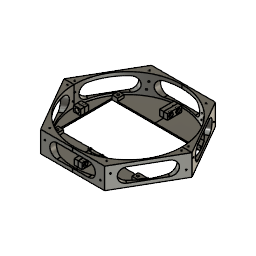
BoTech.StarClock.Top (Autodesk Fusion 360 design; units mm, degrees)
Autodesk Fusion 360 part; units mm, degrees
sketch "Skizze1" plane through (0, 0, 0) normal (0, 0, 1) x (1, 0, 0)
  line L0 (-60.5, 38) -> (60.5, 38)
  line L1 (60.5, 38) -> (60.5, -38)
  line L2 (60.5, -38) -> (-60.5, -38)
  line L3 (-60.5, -38) -> (-60.5, 38)
  line L4 (90, 0.0418) -> (44.9638, 77.9632)
  line L5 (44.9638, 77.9632) -> (-45.0362, 77.9214)
  line L6 (-45.0362, 77.9214) -> (-90, -0.0418)
  line L7 (-90, -0.0418) -> (-44.9638, -77.9632)
  line L8 (-44.9638, -77.9632) -> (45.0362, -77.9214)
  line L9 (45.0362, -77.9214) -> (90, 0.0418)
  line L10 (-0.0205, 160) -> (-138.5743, 79.9822)
  line L11 (-138.5743, 79.9822) -> (-138.5538, -80.0178)
  line L12 (-138.5538, -80.0178) -> (0.0205, -160)
  line L13 (0.0205, -160) -> (138.5743, -79.9822)
  line L14 (138.5743, -79.9822) -> (138.5538, 80.0178)
  line L15 (138.5538, 80.0178) -> (-0.0205, 160)
  line L16 (-45.0362, 77.9214) -> (-0.0205, 160)
  line L17 (-0.0205, 160) -> (44.9638, 77.9632)
  line L18 (44.9638, 77.9632) -> (138.5538, 80.0178)
  line L19 (138.5538, 80.0178) -> (90, 0.0418)
  line L20 (90, 0.0418) -> (138.5743, -79.9822)
  line L21 (138.5743, -79.9822) -> (45.0362, -77.9214)
  line L22 (-44.9638, -77.9632) -> (0.0205, -160)
  line L23 (0.0205, -160) -> (45.0362, -77.9214)
  line L24 (-90, -0.0418) -> (-138.5538, -80.0178)
  line L25 (-138.5538, -80.0178) -> (-44.9638, -77.9632)
  line L26 (-138.5743, 79.9822) -> (-90, -0.0418)
  line L27 (-45.0362, 77.9214) -> (-138.5743, 79.9822)
  circle A0 centre (0, 0) radius 75.8906
  circle A1 centre (-40, 70) radius 1
  circle A2 centre (-80, 5) radius 1
  circle A3 centre (-80, -5) radius 1
  circle A4 centre (40, 70) radius 1
  circle A5 centre (80, 5) radius 1
  circle A6 centre (80, -5) radius 1
  circle A7 centre (-40, -70) radius 1
  circle A8 centre (40, -70) radius 1
  circle A9 centre (0, -45) radius 4
  line L28 (4, -45) -> (6, -45)
  line L29 (-4, -45) -> (-6, -45)
  circle A10 centre (8.25, -45) radius 1
  circle A11 centre (8.25, -45) radius 2.25
  circle A12 centre (-8.2553, -45) radius 1
  circle A13 centre (-8.2553, -45) radius 2.25
  circle A14 centre (0, -45) radius 4
  line L30 (-4, -45) -> (-6, -45)
  line L31 (4, -45) -> (6, -45)
  line L32 (0, 0) -> (-60.5, 0)
  line L33 (-60.5, 0) -> (-60.5, 38)
  line L34 (60.5, -38) -> (52.5, -38)
  line L35 (52.5, -38) -> (52.5, -47)
  line L36 (52.5, -47) -> (60.5, -47)
  line L37 (60.5, -47) -> (60.5, -38)
  line L38 (-60.5, -38) -> (-52.5, -38)
  line L39 (-52.5, -38) -> (-52.5, -47)
  line L40 (-52.5, -47) -> (-60.5, -47)
  line L41 (-60.5, -47) -> (-60.5, -38)
  line L42 (60.5, 38) -> (52.5, 38)
  line L43 (52.5, 38) -> (52.5, 47)
  line L44 (52.5, 47) -> (60.5, 47)
  line L45 (60.5, 47) -> (60.5, 38)
  line L46 (-60.5, 38) -> (-52.5, 38)
  line L47 (-52.5, 38) -> (-52.5, 47)
  line L48 (-52.5, 47) -> (-60.5, 47)
  line L49 (-60.5, 47) -> (-60.5, 38)
  circle A15 centre (56.5, -42.5) radius 1.5
  line L50 (60.5, -38) -> (56.5, -38) construction
  line L51 (56.5, -38) -> (56.5, -42.5) construction
  line L52 (-52.5, -38) -> (-56.5, -38) construction
  line L53 (-56.5, -38) -> (-56.5, -42.5) construction
  circle A16 centre (-56.5, -42.5) radius 1.5
  line L54 (60.5, 47) -> (56.5, 47) construction
  line L55 (56.5, 47) -> (56.5, 42.5) construction
  line L56 (-52.5, 47) -> (-56.5, 47) construction
  line L57 (-56.5, 47) -> (-56.5, 42.5) construction
  circle A17 centre (56.5, 42.5) radius 1.5
  circle A18 centre (-56.5, 42.5) radius 1.5
  circle A19 centre (-56.5, -42.5) radius 2.75
  circle A20 centre (56.5, -42.5) radius 2.75
  circle A21 centre (56.5, 42.5) radius 2.75
  circle A22 centre (-56.5, 42.5) radius 2.75
  line L58 (60.5, -38) -> (65.6915, -38)
  line L59 (60.5, 38) -> (65.6915, 38)
  dimension "d1" = 121
  dimension "d2" = 76
  dimension "d26" = 90
  dimension "d43" = 160
  dimension "d258" = 2
  dimension "d259" = 2
  dimension "d260" = 2
  dimension "d261" = 2
  dimension "d262" = 2
  dimension "d263" = 2
  dimension "d264" = 2
  dimension "d265" = 2
  dimension "d322" = 8
  dimension "d323" = 2
  dimension "d324" = 2
  dimension "d325" = 2
  dimension "d326" = 4.5
  dimension "d327" = 2
  dimension "d328" = 4.5
  dimension "d331" = 8
  dimension "d332" = 2
  dimension "d333" = 2
  dimension "d350" = 60.5
  dimension "d351" = 38
  dimension "d352" = 8
  dimension "d353" = 9
  dimension "d354" = 8
  dimension "d355" = 9
  dimension "d356" = 8
  dimension "d357" = 9
  dimension "d358" = 8
  dimension "d359" = 9
  dimension "d362" = 3
  dimension "d363" = 4
  dimension "d364" = 4.5
  dimension "d365" = 4
  dimension "d366" = 4.5
  dimension "d367" = 3
  dimension "d368" = 4
  dimension "d369" = 4.5
  dimension "d370" = 4
  dimension "d371" = 4.5
  dimension "d372" = 3
  dimension "d373" = 3
  dimension "d376" = 5.5
  dimension "d377" = 5.5
  dimension "d378" = 5.5
  dimension "d379" = 5.5
  constraint horizontal L0
  constraint vertical L1
  constraint horizontal L2
  constraint vertical L3
  constraint coincident A0.centre L32.start
  constraint coincident A9 L28.start
  constraint parallel L2 L28
  constraint coincident A9 L29.start
  constraint parallel L2 L29
  constraint concentric A10 A11
  constraint coincident L28.end A11
  constraint concentric A12 A13
  constraint coincident L28.start A14
  constraint coincident L29.start A14
  constraint perpendicular L3 L32
  constraint perpendicular L32 L33
  constraint horizontal L34
  constraint vertical L35
  constraint horizontal L36
  constraint vertical L37
  constraint horizontal L38
  constraint vertical L39
  constraint horizontal L40
  constraint vertical L41
  constraint horizontal L42
  constraint vertical L43
  constraint horizontal L44
  constraint vertical L45
  constraint horizontal L46
  constraint vertical L47
  constraint horizontal L48
  constraint vertical L49
  constraint midpoint L34 L50.end
  constraint coincident A15.centre L51.end
  constraint coincident L53.end A16.centre
  constraint coincident L55.end A17.centre
  constraint coincident L57.end A18.centre
  constraint concentric A16 A19
  constraint concentric A15 A20
  constraint concentric A17 A21
  constraint concentric A18 A22
  constraint perpendicular L1 L58
  constraint coincident A0 L58.end
  constraint perpendicular L45 L59
  constraint coincident A0 L59.end
  measures "d1" distance of L0.end L0.start
  measures "d2" distance of L2.end L0.start
  measures "d26" distance of L4.start A0.centre
  measures "d43" distance of L10.start A0.centre
  measures "d258" diameter of A1
  measures "d259" diameter of A2
  measures "d260" diameter of A3
  measures "d261" diameter of A4
  measures "d262" diameter of A5
  measures "d263" diameter of A6
  measures "d264" diameter of A7
  measures "d265" diameter of A8
  measures "d322" diameter of A9
  measures "d323" distance of L28.start L28.end
  measures "d324" distance of L29.start L29.end
  measures "d325" diameter of A10
  measures "d326" diameter of A11
  measures "d327" diameter of A12
  measures "d328" diameter of A13
  measures "d331" diameter of A14
  measures "d332" distance of L28.start L28.end
  measures "d333" distance of L29.end L29.start
  measures "d350" distance of A0.centre L32.end
  measures "d351" distance of L32.end L0.start
  measures "d352" distance of L1.end L34.end
  measures "d353" distance of L1.end L36.end
  measures "d354" distance of L2.end L38.end
  measures "d355" distance of L2.end L40.end
  measures "d356" distance of L0.end L42.end
  measures "d357" distance of L0.end L44.end
  measures "d358" distance of L0.start L46.end
  measures "d359" distance of L0.start L48.end
  measures "d362" diameter of A15
  measures "d363" distance of L1.end L50.end
  measures "d364" distance of L50.end A15.centre
  measures "d365" distance of L38.end L52.end
  measures "d366" distance of L53.end L52.end
  measures "d367" diameter of A16
  measures "d368" distance of L44.end L54.end
  measures "d369" distance of L55.end L54.end
  measures "d370" distance of L47.end L56.end
  measures "d371" distance of L57.end L56.end
  measures "d372" diameter of A17
  measures "d373" diameter of A18
  measures "d376" diameter of A19
  measures "d377" diameter of A20
  measures "d378" diameter of A21
  measures "d379" diameter of A22
extrude "Extrusion1" add sketch "Skizze1" along normal blind 30 contours A0 L48 L49 | A0 L40 L41 | A0 L44 L45 | A0 L36 L37 | L4 L5 L6 L7 L8 L9 makes body 1
extrude "Extrusion2" add sketch "Skizze1" along normal blind 2 contours L0 A0 L46 L47 L48 L49 | L3 A0 L33 L41 L49 | L0 A0 L43 L44 L47 L48 | L0 A0 L42 L43 L44 L45 | L2 A0 L38 L39 L40 L41 | A0 L45 L59 | L2 A0 L35 L36 L39 L40 | L2 A0 L34 L35 L36 L37 | A0 L37 L58 | A1 | A2 | A3 | A4 | A5 | A6 | A7 | A8 | A10 | A11 | A12 | A13 | A19 | A20 | A21 | A22 bodies 1
extrude "Extrusion27" add sketch "Skizze1" along normal blind 8 contours A11 | A13 bodies 1
sketch "Skizze2" plane through (0.0362, -77.9423, 0) normal (0.000464, -1, 0) x (1, 0.000464, 0)
  line L0 (-45, 0) -> (45, 0)
  line L1 (45, 0) -> (45, 30)
  line L2 (-45, 30) -> (-45, 0)
  line L3 (-22, 25) -> (22, 25)
  line L4 (22, 25) -> (22, 5)
  line L5 (22, 5) -> (-22, 5)
  arc A0 (-22, 25) -> (-22, 5) centre (-22, 15) ccw
  arc A1 (22, 5) -> (22, 25) centre (22, 15) ccw
  circle A2 centre (39, 10) radius 3.5
  circle A3 centre (39, 10) radius 1
  circle A4 centre (39, 10) radius 2.5
  line L6 (-45, 30) -> (45, 30)
  line L7 (45, 30) -> (45, 0)
  line L8 (45, 0) -> (-45, 0)
  line L9 (-45, 0) -> (-45, 30)
  line L10 (45, 15) -> (39, 15)
  line L11 (39, 15) -> (22, 15)
  line L12 (22, 15) -> (-22, 15)
  line L13 (-22, 15) -> (-39, 15)
  line L14 (-39, 15) -> (-45, 15)
  circle A5 centre (-39, 20) radius 3.5
  circle A6 centre (-39, 20) radius 1
  circle A7 centre (-39, 20) radius 2.5
  line L15 (-39, 15) -> (-39, 20)
  line L16 (39, 15) -> (39, 10)
  point P0 (-57.5, 15)
  point P1 (-39, 20)
  dimension "d109" = 2
  dimension "d110" = 5
  dimension "d111" = 6
  dimension "d112" = 17
  dimension "d113" = 44
  dimension "d114" = 17
  dimension "d115" = 6
  dimension "d161" = 2
  dimension "d162" = 5
  dimension "d163" = 5
  dimension "d165" = 5
  constraint perpendicular L4 L5
  constraint tangent L3 A0
  constraint tangent L5 A1
  constraint concentric A3 A4
  constraint concentric A2 A4
  constraint horizontal L6
  constraint vertical L7
  constraint horizontal L8
  constraint vertical L9
  constraint coincident L0.end L1.start
  constraint coincident L2.start L6.start
  constraint midpoint L7 L10.start
  constraint perpendicular L7 L10
  constraint parallel L10 L11
  constraint perpendicular L4 L12
  constraint perpendicular L9 L14
  constraint concentric A6 A7
  constraint concentric A5 A7
  constraint coincident P1 A5.centre
  constraint perpendicular L13 L15
  constraint perpendicular L10 L16
  constraint coincident A2.centre A3.centre
  measures "d109" diameter of A3
  measures "d110" diameter of A4
  measures "d111" distance of L10.start L10.end
  measures "d112" distance of L10.end A1.centre
  measures "d113" distance of A1.centre A0.centre
  measures "d114" distance of A0.centre L13.end
  measures "d115" distance of L13.end L14.end
  measures "d161" diameter of A6
  measures "d162" diameter of A7
  measures "d163" distance of L13.end P1
  measures "d165" distance of L10.end A2.centre
sketch "Skizze3" plane through (67.5181, -38.9398, 0) normal (0.866257, -0.499598, 0) x (0.499598, 0.866257, 0)
  circle A0 centre (-39, 20) radius 3.5
  line L0 (22, 15) -> (-22, 15)
  circle A1 centre (-39, 20) radius 2.5
  line L1 (22, 5) -> (-22, 5)
  line L2 (-22, 25) -> (22, 25)
  line L3 (45, 0) -> (45, 30)
  line L4 (-39, 15) -> (-45, 15)
  line L5 (22, 25) -> (22, 5)
  line L6 (-45, 0) -> (-45, 30)
  line L7 (-45, 30) -> (-45, 0)
  line L8 (-45, 0) -> (45, 0)
  line L9 (-22, 15) -> (-39, 15)
  line L10 (-45, 30) -> (45, 30)
  line L11 (39, 15) -> (22, 15)
  line L12 (45, 30) -> (45, 0)
  line L13 (-39, 15) -> (-39, 20)
  arc A2 (22, 5) -> (22, 25) centre (22, 15) ccw
  circle A3 centre (-39, 20) radius 1
  circle A4 centre (39, 10) radius 3.5
  line L14 (45, 15) -> (39, 15)
  line L15 (39, 15) -> (39, 10)
  circle A5 centre (39, 10) radius 2.5
  line L16 (45, 0) -> (-45, 0)
  circle A6 centre (39, 10) radius 1
  arc A7 (-22, 25) -> (-22, 5) centre (-22, 15) ccw
  point P0 (-39, 20)
  dimension "d166" = 2
  dimension "d167" = 5
  dimension "d168" = 6
  dimension "d169" = 17
  dimension "d170" = 44
  dimension "d171" = 17
  dimension "d172" = 6
  dimension "d173" = 2
  dimension "d174" = 5
  dimension "d175" = 5
  dimension "d176" = 5
  constraint perpendicular L1 L5
  constraint tangent L2 A7
  constraint tangent L1 A2
  constraint concentric A5 A6
  constraint concentric A4 A5
  constraint horizontal L10
  constraint vertical L12
  constraint horizontal L16
  constraint vertical L6
  constraint coincident L3.start L8.end
  constraint coincident L6.end L7.start
  constraint midpoint L14.start L12
  constraint perpendicular L12 L14
  constraint parallel L11 L14
  constraint perpendicular L0 L5
  constraint perpendicular L4 L6
  constraint concentric A1 A3
  constraint concentric A0 A1
  constraint coincident P0 A0.centre
  constraint perpendicular L9 L13
  constraint perpendicular L14 L15
  constraint coincident A4.centre L15.end
  measures "d166" diameter of A6
  measures "d167" diameter of A5
  measures "d168" distance of L11.start L14.start
  measures "d169" distance of L0.start L11.start
  measures "d170" distance of L0.start L0.end
  measures "d171" distance of L0.end L4.start
  measures "d172" distance of L4.end L4.start
  measures "d173" diameter of A3
  measures "d174" diameter of A1
  measures "d175" distance of P0 L4.start
  measures "d176" distance of L11.start A4.centre
sketch "Skizze4" plane through (67.4819, 39.0025, 0) normal (0.865793, 0.500402, 0) x (-0.500402, 0.865793, 0)
  circle A0 centre (-39, 20) radius 3.5
  line L0 (22, 15) -> (-22, 15)
  circle A1 centre (-39, 20) radius 2.5
  line L1 (22, 5) -> (-22, 5)
  line L2 (-22, 25) -> (22, 25)
  line L3 (45, 0) -> (45, 30)
  line L4 (-39, 15) -> (-45, 15)
  line L5 (22, 25) -> (22, 5)
  line L6 (-45, 0) -> (-45, 30)
  line L7 (-45, 30) -> (-45, 0)
  line L8 (-45, 0) -> (45, 0)
  line L9 (-22, 15) -> (-39, 15)
  line L10 (-45, 30) -> (45, 30)
  line L11 (39, 15) -> (22, 15)
  line L12 (45, 30) -> (45, 0)
  line L13 (-39, 15) -> (-39, 20)
  arc A2 (22, 5) -> (22, 25) centre (22, 15) ccw
  circle A3 centre (-39, 20) radius 1
  circle A4 centre (39, 10) radius 3.5
  line L14 (45, 15) -> (39, 15)
  line L15 (39, 15) -> (39, 10)
  circle A5 centre (39, 10) radius 2.5
  line L16 (45, 0) -> (-45, 0)
  circle A6 centre (39, 10) radius 1
  arc A7 (-22, 25) -> (-22, 5) centre (-22, 15) ccw
  point P0 (-39, 20)
  dimension "d177" = 2
  dimension "d178" = 5
  dimension "d179" = 6
  dimension "d180" = 17
  dimension "d181" = 44
  dimension "d182" = 17
  dimension "d183" = 6
  dimension "d184" = 2
  dimension "d185" = 5
  dimension "d186" = 5
  dimension "d187" = 5
  constraint perpendicular L1 L5
  constraint tangent L2 A7
  constraint tangent L1 A2
  constraint concentric A5 A6
  constraint concentric A4 A5
  constraint horizontal L10
  constraint vertical L12
  constraint horizontal L16
  constraint vertical L6
  constraint coincident L3.start L8.end
  constraint coincident L6.end L7.start
  constraint midpoint L14.start L12
  constraint perpendicular L12 L14
  constraint parallel L11 L14
  constraint perpendicular L0 L5
  constraint perpendicular L4 L6
  constraint concentric A1 A3
  constraint concentric A0 A1
  constraint coincident P0 A0.centre
  constraint perpendicular L9 L13
  constraint perpendicular L14 L15
  constraint coincident A4.centre L15.end
  measures "d177" diameter of A6
  measures "d178" diameter of A5
  measures "d179" distance of L11.start L14.start
  measures "d180" distance of L0.start L11.start
  measures "d181" distance of L0.start L0.end
  measures "d182" distance of L0.end L4.start
  measures "d183" distance of L4.end L4.start
  measures "d184" diameter of A3
  measures "d185" diameter of A1
  measures "d186" distance of P0 L4.start
  measures "d187" distance of L11.start A4.centre
sketch "Skizze5" plane through (-0.0362, 77.9423, 0) normal (-0.000464, 1, 0) x (-1, -0.000464, 0)
  circle A0 centre (-39, 20) radius 3.5
  line L0 (22, 15) -> (-22, 15)
  circle A1 centre (-39, 20) radius 2.5
  line L1 (22, 5) -> (-22, 5)
  line L2 (-22, 25) -> (22, 25)
  line L3 (45, 0) -> (45, 30)
  line L4 (-39, 15) -> (-45, 15)
  line L5 (22, 25) -> (22, 5)
  line L6 (-45, 0) -> (-45, 30)
  line L7 (-45, 30) -> (-45, 0)
  line L8 (-45, 0) -> (45, 0)
  line L9 (-22, 15) -> (-39, 15)
  line L10 (-45, 30) -> (45, 30)
  line L11 (39, 15) -> (22, 15)
  line L12 (45, 30) -> (45, 0)
  line L13 (-39, 15) -> (-39, 20)
  arc A2 (22, 5) -> (22, 25) centre (22, 15) ccw
  circle A3 centre (-39, 20) radius 1
  circle A4 centre (39, 10) radius 3.5
  line L14 (45, 15) -> (39, 15)
  line L15 (39, 15) -> (39, 10)
  circle A5 centre (39, 10) radius 2.5
  line L16 (45, 0) -> (-45, 0)
  circle A6 centre (39, 10) radius 1
  arc A7 (-22, 25) -> (-22, 5) centre (-22, 15) ccw
  point P0 (-39, 20)
  dimension "d188" = 2
  dimension "d189" = 5
  dimension "d190" = 6
  dimension "d191" = 17
  dimension "d192" = 44
  dimension "d193" = 17
  dimension "d194" = 6
  dimension "d195" = 2
  dimension "d196" = 5
  dimension "d197" = 5
  dimension "d198" = 5
  constraint perpendicular L1 L5
  constraint tangent L2 A7
  constraint tangent L1 A2
  constraint concentric A5 A6
  constraint concentric A4 A5
  constraint horizontal L10
  constraint vertical L12
  constraint horizontal L16
  constraint vertical L6
  constraint coincident L3.start L8.end
  constraint coincident L6.end L7.start
  constraint midpoint L14.start L12
  constraint perpendicular L12 L14
  constraint parallel L11 L14
  constraint perpendicular L0 L5
  constraint perpendicular L4 L6
  constraint concentric A1 A3
  constraint concentric A0 A1
  constraint coincident P0 A0.centre
  constraint perpendicular L9 L13
  constraint perpendicular L14 L15
  constraint coincident A4.centre L15.end
  measures "d188" diameter of A6
  measures "d189" diameter of A5
  measures "d190" distance of L11.start L14.start
  measures "d191" distance of L0.start L11.start
  measures "d192" distance of L0.start L0.end
  measures "d193" distance of L0.end L4.start
  measures "d194" distance of L4.end L4.start
  measures "d195" diameter of A3
  measures "d196" diameter of A1
  measures "d197" distance of P0 L4.start
  measures "d198" distance of L11.start A4.centre
sketch "Skizze6" plane through (-67.5181, 38.9398, 0) normal (-0.866257, 0.499598, 0) x (-0.499598, -0.866257, 0)
  circle A0 centre (-39, 20) radius 3.5
  line L0 (22, 15) -> (-22, 15)
  circle A1 centre (-39, 20) radius 2.5
  line L1 (22, 5) -> (-22, 5)
  line L2 (-22, 25) -> (22, 25)
  line L3 (45, 0) -> (45, 30)
  line L4 (-39, 15) -> (-45, 15)
  line L5 (22, 25) -> (22, 5)
  line L6 (-45, 0) -> (-45, 30)
  line L7 (-45, 30) -> (-45, 0)
  line L8 (-45, 0) -> (45, 0)
  line L9 (-22, 15) -> (-39, 15)
  line L10 (-45, 30) -> (45, 30)
  line L11 (39, 15) -> (22, 15)
  line L12 (45, 30) -> (45, 0)
  line L13 (-39, 15) -> (-39, 20)
  arc A2 (22, 5) -> (22, 25) centre (22, 15) ccw
  circle A3 centre (-39, 20) radius 1
  circle A4 centre (39, 10) radius 3.5
  line L14 (45, 15) -> (39, 15)
  line L15 (39, 15) -> (39, 10)
  circle A5 centre (39, 10) radius 2.5
  line L16 (45, 0) -> (-45, 0)
  circle A6 centre (39, 10) radius 1
  arc A7 (-22, 25) -> (-22, 5) centre (-22, 15) ccw
  point P0 (-39, 20)
  dimension "d199" = 2
  dimension "d200" = 5
  dimension "d201" = 6
  dimension "d202" = 17
  dimension "d203" = 44
  dimension "d204" = 17
  dimension "d205" = 6
  dimension "d206" = 2
  dimension "d207" = 5
  dimension "d208" = 5
  dimension "d209" = 5
  constraint perpendicular L1 L5
  constraint tangent L2 A7
  constraint tangent L1 A2
  constraint concentric A5 A6
  constraint concentric A4 A5
  constraint horizontal L10
  constraint vertical L12
  constraint horizontal L16
  constraint vertical L6
  constraint coincident L3.start L8.end
  constraint coincident L6.end L7.start
  constraint midpoint L14.start L12
  constraint perpendicular L12 L14
  constraint parallel L11 L14
  constraint perpendicular L0 L5
  constraint perpendicular L4 L6
  constraint concentric A1 A3
  constraint concentric A0 A1
  constraint coincident P0 A0.centre
  constraint perpendicular L9 L13
  constraint perpendicular L14 L15
  constraint coincident A4.centre L15.end
  measures "d199" diameter of A6
  measures "d200" diameter of A5
  measures "d201" distance of L11.start L14.start
  measures "d202" distance of L0.start L11.start
  measures "d203" distance of L0.start L0.end
  measures "d204" distance of L0.end L4.start
  measures "d205" distance of L4.end L4.start
  measures "d206" diameter of A3
  measures "d207" diameter of A1
  measures "d208" distance of P0 L4.start
  measures "d209" distance of L11.start A4.centre
sketch "Skizze7" plane through (-67.4819, -39.0025, 0) normal (-0.865793, -0.500402, 0) x (0.500402, -0.865793, 0)
  circle A0 centre (-39, 20) radius 3.5
  line L0 (22, 15) -> (-22, 15)
  circle A1 centre (-39, 20) radius 2.5
  line L1 (22, 5) -> (-22, 5)
  line L2 (-22, 25) -> (22, 25)
  line L3 (45, 0) -> (45, 30)
  line L4 (-39, 15) -> (-45, 15)
  line L5 (22, 25) -> (22, 5)
  line L6 (-45, 0) -> (-45, 30)
  line L7 (-45, 30) -> (-45, 0)
  line L8 (-45, 0) -> (45, 0)
  line L9 (-22, 15) -> (-39, 15)
  line L10 (-45, 30) -> (45, 30)
  line L11 (39, 15) -> (22, 15)
  line L12 (45, 30) -> (45, 0)
  line L13 (-39, 15) -> (-39, 20)
  arc A2 (22, 5) -> (22, 25) centre (22, 15) ccw
  circle A3 centre (-39, 20) radius 1
  circle A4 centre (39, 10) radius 3.5
  line L14 (45, 15) -> (39, 15)
  line L15 (39, 15) -> (39, 10)
  circle A5 centre (39, 10) radius 2.5
  line L16 (45, 0) -> (-45, 0)
  circle A6 centre (39, 10) radius 1
  arc A7 (-22, 25) -> (-22, 5) centre (-22, 15) ccw
  point P0 (-39, 20)
  dimension "d210" = 2
  dimension "d211" = 5
  dimension "d212" = 6
  dimension "d213" = 17
  dimension "d214" = 44
  dimension "d215" = 17
  dimension "d216" = 6
  dimension "d217" = 2
  dimension "d218" = 5
  dimension "d219" = 5
  dimension "d220" = 5
  constraint perpendicular L1 L5
  constraint tangent L2 A7
  constraint tangent L1 A2
  constraint concentric A5 A6
  constraint concentric A4 A5
  constraint horizontal L10
  constraint vertical L12
  constraint horizontal L16
  constraint vertical L6
  constraint coincident L3.start L8.end
  constraint coincident L6.end L7.start
  constraint midpoint L14.start L12
  constraint perpendicular L12 L14
  constraint parallel L11 L14
  constraint perpendicular L0 L5
  constraint perpendicular L4 L6
  constraint concentric A1 A3
  constraint concentric A0 A1
  constraint coincident P0 A0.centre
  constraint perpendicular L9 L13
  constraint perpendicular L14 L15
  constraint coincident A4.centre L15.end
  measures "d210" diameter of A6
  measures "d211" diameter of A5
  measures "d212" distance of L11.start L14.start
  measures "d213" distance of L0.start L11.start
  measures "d214" distance of L0.start L0.end
  measures "d215" distance of L0.end L4.start
  measures "d216" distance of L4.end L4.start
  measures "d217" diameter of A3
  measures "d218" diameter of A1
  measures "d219" distance of P0 L4.start
  measures "d220" distance of L11.start A4.centre
extrude "Extrusion3" cut sketch "Skizze2" against normal blind 28 contours L4 L5 A0 L12 L13 | L3 L4 A0 L12 L13 | L4 A1 L11 | L4 A1 L11 | A3 | A6 bodies 1
extrude "Extrusion4" cut sketch "Skizze7" against normal blind 28 contours L0 L1 L5 L9 A7 | L0 L2 L5 L9 A7 | L5 L11 A2 | L5 L11 A2 | A3 | A6 bodies 1
extrude "Extrusion5" cut sketch "Skizze6" against normal blind 28 contours L0 L1 L5 L9 A7 | L0 L2 L5 L9 A7 | L5 L11 A2 | L5 L11 A2 | A3 | A6 bodies 1
extrude "Extrusion6" cut sketch "Skizze5" against normal blind 28 contours L0 L1 L5 L9 A7 | L0 L2 L5 L9 A7 | L5 L11 A2 | L5 L11 A2 | A3 | A6 bodies 1
extrude "Extrusion7" cut sketch "Skizze4" against normal blind 28 contours L0 L1 L5 L9 A7 | L0 L2 L5 L9 A7 | L5 L11 A2 | L5 L11 A2 | A3 | A6 bodies 1
extrude "Extrusion8" cut sketch "Skizze3" against normal blind 28 contours L0 L1 L5 L9 A7 | L0 L2 L5 L9 A7 | L5 L11 A2 | L5 L11 A2 | A3 | A6 bodies 1
extrude "Extrusion28" cut sketch "Skizze1" along normal blind 3 from surface at 2 contours A0 L48 L49 | A0 L40 L41 | A0 L44 L45 | A0 L36 L37 bodies 1
extrude "Extrusion29" add sketch "Skizze1" along normal blind 6 contours L0 A0 L46 L47 L48 L49 | A0 L48 L49 | L0 A0 L42 L43 L44 L45 | L2 A0 L38 L39 L40 L41 | A0 L40 L41 | A0 L45 L59 | A0 L44 L45 | L2 A0 L34 L35 L36 L37 | A0 L37 L58 | A0 L36 L37 | A19 | A20 | A21 | A22 bodies 1
extrude "Extrusion30" cut sketch "Skizze1" along normal blind 4 contours A19 | A20 | A21 | A22 bodies 1
sketch "Skizze19" plane through (0, -38, 0) normal (0, 1, 0) x (-1, 0, 0)
  line L0 (-65.6915, 0) -> (60.5, 0)
  line L1 (60.5, 0) -> (60.5, 2)
  line L2 (60.5, 2) -> (60.5, 6)
  line L3 (60.5, 6) -> (52.5, 6)
  line L4 (52.5, 6) -> (52.5, 2)
  line L5 (52.5, 2) -> (-52.5, 2)
  line L6 (-52.5, 2) -> (-52.5, 6)
  line L7 (-52.5, 6) -> (-65.6915, 6)
  line L8 (-65.6915, 6) -> (-65.6915, 5)
  line L9 (-65.6915, 5) -> (-65.6915, 0)
  line L10 (-60.5, 0) -> (-60.5, 6)
  line L11 (-65.6915, 6) -> (-52.5, 6)
  line L12 (-52.5, 6) -> (-52.5, 0)
  line L13 (-52.5, 0) -> (-65.6915, 0)
  line L14 (-65.6915, 0) -> (-65.6915, 6)
  circle A0 centre (-63.0958, 3) radius 1
  line L15 (-60.5, 3) -> (-65.6915, 3)
  circle A1 centre (-63.0958, 3) radius 1.5
  line L16 (-61.5958, 3) -> (-61.0958, 3)
  line L17 (-63.0958, 4.5) -> (-63.0958, 5)
  line L18 (-61.1, 5) -> (-65.1, 5)
  line L19 (-65.1, 5) -> (-65.1, 1)
  line L20 (-65.1, 1) -> (-63, 1)
  line L21 (-61.1, 2.9) -> (-61.1, 5)
  arc A2 (-63, 1) -> (-61.1, 2.9) centre (-63, 2.9) ccw
  point P0 (-61.1, 1)
  dimension "d382" = 2
  dimension "d383" = 5.1915
  dimension "d386" = 3
  dimension "d387" = 0.5
  dimension "d388" = 0.5
  dimension "d389" = 4
  dimension "d390" = 4
  dimension "d391" = 1.9
  constraint coincident L0 L10.start
  constraint coincident L7 L10.end
  constraint perpendicular L7 L10
  constraint horizontal L11
  constraint vertical L12
  constraint horizontal L13
  constraint vertical L14
  constraint coincident L0 L12.end
  constraint coincident L7.end L8.start
  constraint midpoint L10 L15.start
  constraint midpoint L14 L15.end
  constraint midpoint A0.centre L15
  constraint concentric A0 A1
  constraint coincident L15 L16.start
  constraint coincident A1 L16.start
  constraint coincident L15 L16.end
  constraint coincident A1 L17.start
  constraint perpendicular L15 L17
  constraint horizontal L18
  constraint vertical L19
  constraint horizontal L20
  constraint vertical L21
  constraint coincident P0 L21
  constraint coincident P0 L20
  constraint tangent L21 A2
  constraint tangent L20 A2
  measures "d382" diameter of A0
  measures "d383" distance of L15.start L15.end
  measures "d386" diameter of A1
  measures "d387" distance of L16.start L16.end
  measures "d388" distance of L17.start L17.end
  measures "d389" distance of L18.start L18.end
  measures "d390" distance of L18.start P0
  measures "d391" radius of A2
extrude "Extrusion31" add sketch "Skizze19" along normal blind 3 contours A0 L15 | A0 L15 bodies 1
extrude "Extrusion32" add sketch "Skizze19" along normal blind 3 from surface at 73 contours A0 L15 | A0 L15 bodies 1
sketch "Skizze8" plane through (0, 0, 2) normal (0, 0, 1) x (-1, 0, 0)
  line L0 (0, -20) -> (0, 10)
  line L1 (5.5, 70) -> (-5.5, 70)
  line L2 (-5.5, 70) -> (-5.5, 50)
  line L3 (-5.5, 50) -> (5.5, 50)
  line L4 (5.5, 50) -> (5.5, 70)
  line L5 (15, -0.0337) -> (-20, -0.0337)
  line L6 (61, 5.5) -> (71, 5.5)
  line L7 (71, 5.5) -> (71, -5.5)
  line L8 (61, -5.5) -> (61, 5.5)
  line L9 (71, -5.5) -> (61, -5.5)
  line L10 (-45.0362, 77.9214) -> (-90, -0.0418)
  line L11 (-90, -0.0418) -> (-44.9638, -77.9632)
  line L12 (5.5, -70.0674) -> (-5.5, -70.0674)
  line L13 (-5.5, -70.0674) -> (-5.5, -50.0674)
  line L14 (5.5, -50.0674) -> (5.5, -70.0674)
  line L15 (-5.5, -50.0674) -> (5.5, -50.0674)
  circle A0 centre (-40, 70) radius 1
  circle A1 centre (40, -70) radius 1
  circle A2 centre (80, -5) radius 1
  circle A3 centre (-40, -70) radius 1
  circle A4 centre (40, 70) radius 1
  circle A5 centre (-80, 5) radius 1
  circle A6 centre (-8.25, 45) radius 1
  circle A7 centre (80, 5) radius 1
  circle A8 centre (-80, -5) radius 1
  circle A9 centre (8.2553, 45) radius 1
  dimension "d101" = 11
  dimension "d102" = 20
  constraint vertical L0
  constraint horizontal L1
  constraint vertical L2
  constraint horizontal L3
  constraint vertical L4
  constraint perpendicular L0 L5
  constraint symmetric L1.start L5 L12.start
  constraint symmetric L1.end L5 L12.end
  constraint symmetric L2.end L5 L13.end
  constraint symmetric L3.end L5 L14.start
  measures "d101" distance of L1.start L1.end
  measures "d102" distance of L1.start L3.end
extrude "Extrusion9" add sketch "Skizze8" along normal blind 8 contours L1 L2 L3 L4 | L6 L7 L8 L9 | L12 L13 L14 L15 bodies 1
sketch "Skizze11" plane through (0, -5.5, 0) normal (0, -1, 0) x (1, 0, 0)
  line L0 (-71, 2) -> (-61, 2)
  line L1 (-61, 2) -> (-61, 10)
  line L2 (-71, 10) -> (-71, 2)
  line L3 (0, 0) -> (0, 20)
  line L4 (71, 12) -> (71, 2)
  line L5 (71, 2) -> (61, 2)
  line L6 (61, 2) -> (61, 12)
  circle A0 centre (-66, 6) radius 3
  circle A1 centre (-66, 6) radius 1.75
  circle A2 centre (66, 6) radius 1.75
  circle A3 centre (66, 6) radius 3
  constraint coincident L3.start origin
  constraint vertical L3
  constraint symmetric L0.start L3 L4.end
  constraint symmetric L0.end L3 L5.end
  constraint coincident A0.centre A1.centre
  constraint symmetric L3 A0 A3
  constraint symmetric L3 A1 A2
sketch "Skizze12" plane through (-5.5, 0, 0) normal (-1, 0, 0) x (0, -1, 0)
  line L0 (-70.0674, 2) -> (-60.0674, 2)
  line L1 (-60.0674, 2) -> (-60.0674, 10)
  line L2 (-70.0674, 10) -> (-70.0674, 2)
  line L3 (0, 0) -> (0, 20)
  circle A0 centre (-65, 6) radius 3
  circle A1 centre (-65, 6) radius 1.75
  line L4 (-70.0674, 2) -> (-50.0674, 2)
  line L5 (-50.0674, 2) -> (-50.0674, 10)
  line L6 (-50.0674, 10) -> (-70.0674, 10)
  line L7 (-70.0674, 10) -> (-70.0674, 2)
  circle A2 centre (-55, 6) radius 3
  circle A3 centre (-55, 6) radius 1.75
  line L8 (70.0674, 2) -> (50.0674, 2)
  line L9 (50.0674, 2) -> (50.0674, 10)
  line L10 (70.0674, 10) -> (70.0674, 2)
  line L11 (70.0674, 2) -> (60.0674, 2)
  circle A4 centre (65, 6) radius 3
  line L12 (70.0674, 10) -> (70.0674, 2)
  circle A5 centre (55, 6) radius 3
  line L13 (50.0674, 10) -> (70.0674, 10)
  circle A6 centre (65, 6) radius 1.75
  line L14 (60.0674, 2) -> (60.0674, 10)
  circle A7 centre (55, 6) radius 1.75
  constraint coincident L3.start origin
  constraint vertical L3
  constraint symmetric L0.start L3 L8.start
  constraint symmetric L0.end L3 L11.end
  constraint symmetric L1.end L3 L14.end
  constraint symmetric L2.start L3 L10.start
  constraint symmetric L3 A0 A4
  constraint symmetric L3 A1 A6
  constraint symmetric L3 L0.start L8.start
  constraint symmetric L3 L4.end L8.end
  constraint symmetric L3 L5.end L9.end
  constraint symmetric L3 L2.start L10.start
  constraint symmetric L3 A2 A5
  constraint symmetric L3 A3 A7
sketch "Skizze13" plane through (5.5, 0, 0) normal (1, 0, 0) x (0, 1, 0)
  line L0 (60.0674, 2) -> (70.0674, 2)
  line L1 (70.0674, 2) -> (70.0674, 10)
  line L2 (70.0674, 10) -> (60.0674, 10)
  line L3 (60.0674, 10) -> (60.0674, 2)
  line L4 (66.7321, 3) -> (63.2679, 3)
  line L5 (68.4641, 6) -> (66.7321, 3)
  line L6 (66.7321, 9) -> (68.4641, 6)
  line L7 (63.2679, 3) -> (61.5359, 6)
  line L8 (61.5359, 6) -> (63.2679, 9)
  circle A0 centre (65, 6) radius 1.75
  line L9 (63.2679, 9) -> (66.7321, 9)
  line L10 (66.7321, 3) -> (63.2679, 3)
  line L11 (68.4641, 6) -> (66.7321, 3)
  line L12 (66.7321, 9) -> (68.4641, 6)
  line L13 (63.2679, 3) -> (61.5359, 6)
  line L14 (61.5359, 6) -> (63.2679, 9)
  circle A1 centre (65, 6) radius 1.75
  line L15 (63.2679, 9) -> (66.7321, 9)
  line L16 (0, 0) -> (0, 15.511)
  line L17 (50.0674, 2) -> (70.0674, 2)
  line L18 (70.0674, 2) -> (70.0674, 10)
  line L19 (70.0674, 10) -> (50.0674, 10)
  line L20 (50.0674, 10) -> (50.0674, 2)
  line L21 (58.4641, 6) -> (56.7321, 3)
  line L22 (53.2679, 9) -> (56.7321, 9)
  line L23 (56.7321, 3) -> (53.2679, 3)
  line L24 (53.2679, 3) -> (51.5359, 6)
  line L25 (53.2679, 9) -> (56.7321, 9)
  circle A2 centre (55, 6) radius 1.75
  line L26 (56.7321, 9) -> (58.4641, 6)
  line L27 (56.7321, 9) -> (58.4641, 6)
  circle A3 centre (55, 6) radius 1.75
  line L28 (56.7321, 3) -> (53.2679, 3)
  line L29 (58.4641, 6) -> (56.7321, 3)
  line L30 (53.2679, 3) -> (51.5359, 6)
  line L31 (51.5359, 6) -> (53.2679, 9)
  line L32 (51.5359, 6) -> (53.2679, 9)
  line L33 (-53.2679, 3) -> (-51.5359, 6)
  line L34 (-70.0674, 2) -> (-70.0674, 10)
  line L35 (-60.0674, 2) -> (-70.0674, 2)
  line L36 (-63.2679, 3) -> (-61.5359, 6)
  line L37 (-66.7321, 3) -> (-63.2679, 3)
  line L38 (-63.2679, 9) -> (-66.7321, 9)
  line L39 (-50.0674, 2) -> (-70.0674, 2)
  line L40 (-63.2679, 9) -> (-66.7321, 9)
  line L41 (-68.4641, 6) -> (-66.7321, 3)
  circle A4 centre (-55, 6) radius 1.75
  circle A5 centre (-55, 6) radius 1.75
  line L42 (-56.7321, 9) -> (-58.4641, 6)
  line L43 (-51.5359, 6) -> (-53.2679, 9)
  line L44 (-56.7321, 3) -> (-53.2679, 3)
  line L45 (-58.4641, 6) -> (-56.7321, 3)
  line L46 (-53.2679, 9) -> (-56.7321, 9)
  line L47 (-51.5359, 6) -> (-53.2679, 9)
  line L48 (-56.7321, 3) -> (-53.2679, 3)
  line L49 (-61.5359, 6) -> (-63.2679, 9)
  line L50 (-60.0674, 10) -> (-60.0674, 2)
  line L51 (-70.0674, 2) -> (-70.0674, 10)
  line L52 (-63.2679, 3) -> (-61.5359, 6)
  line L53 (-58.4641, 6) -> (-56.7321, 3)
  line L54 (-70.0674, 10) -> (-60.0674, 10)
  line L55 (-66.7321, 3) -> (-63.2679, 3)
  line L56 (-66.7321, 9) -> (-68.4641, 6)
  line L57 (-53.2679, 9) -> (-56.7321, 9)
  circle A6 centre (-65, 6) radius 1.75
  line L58 (-53.2679, 3) -> (-51.5359, 6)
  line L59 (-56.7321, 9) -> (-58.4641, 6)
  line L60 (-50.0674, 10) -> (-50.0674, 2)
  line L61 (-68.4641, 6) -> (-66.7321, 3)
  line L62 (-61.5359, 6) -> (-63.2679, 9)
  circle A7 centre (-65, 6) radius 1.75
  line L63 (-70.0674, 10) -> (-50.0674, 10)
  line L64 (-66.7321, 9) -> (-68.4641, 6)
  point P0 (65, 6)
  point P1 (65, 6)
  point P2 (55, 6)
  point P3 (55, 6)
  point P4 (-55, 6)
  point P5 (-55, 6)
  point P6 (-65, 6)
  point P7 (-65, 6)
  constraint coincident L16.start origin
  constraint vertical L16
  constraint symmetric L0.start L16 L35.start
  constraint symmetric L0.end L16 L34.start
  constraint symmetric L1.end L16 L34.end
  constraint symmetric L2.end L16 L50.start
  constraint symmetric L5.start L16 L41.start
  constraint symmetric L8.end L16 L38.start
  constraint symmetric P1 L16 P6
  constraint symmetric L6.start L16 L38.end
  constraint symmetric L4.end L16 L36.start
  constraint symmetric L4.start L16 L37.start
  constraint symmetric L7.end L16 L36.end
  constraint symmetric A0 L16 A7
  constraint symmetric P1 L16 P7
  constraint symmetric A1 L16 A6
  constraint symmetric L16 L17.start L39.start
  constraint symmetric L16 L0.end L34.start
  constraint symmetric L16 L1.end L34.end
  constraint symmetric L16 L19.end L60.start
  constraint symmetric L16 L21.end L44.start
  constraint symmetric L16 P3 P5
  constraint symmetric L16 L21.start L42.end
  constraint symmetric L16 L23.end L33.start
  constraint symmetric L16 L22.start L43.end
  constraint symmetric L16 L24.end L33.end
  constraint symmetric L16 L22.end L42.start
  constraint symmetric L16 A2 A5
  constraint symmetric L16 A3 A4
sketch "Skizze14" plane through (0, 5.5, 0) normal (0, 1, 0) x (-1, 0, 0)
  line L0 (61, 2) -> (71, 2)
  line L1 (71, 2) -> (71, 10)
  line L2 (71, 10) -> (61, 10)
  line L3 (61, 10) -> (61, 2)
  line L4 (67.7321, 3) -> (64.2679, 3)
  line L5 (69.4641, 6) -> (67.7321, 3)
  line L6 (67.7321, 9) -> (69.4641, 6)
  line L7 (64.2679, 3) -> (62.5359, 6)
  line L8 (62.5359, 6) -> (64.2679, 9)
  circle A0 centre (66, 6) radius 1.75
  line L9 (64.2679, 9) -> (67.7321, 9)
  line L10 (0, 0) -> (0, 20)
  line L11 (-64.2679, 9) -> (-67.7321, 9)
  line L12 (-67.7321, 3) -> (-64.2679, 3)
  line L13 (-62.5359, 6) -> (-64.2679, 9)
  line L14 (-67.7321, 9) -> (-69.4641, 6)
  line L15 (-64.2679, 3) -> (-62.5359, 6)
  circle A1 centre (-66, 6) radius 1.75
  line L16 (-69.4641, 6) -> (-67.7321, 3)
  point P0 (66, 6)
  point P1 (-66, 6)
  constraint symmetric L5.start L10 L14.end
  constraint symmetric L8.end L10 L11.start
  constraint symmetric P0 L10 P1
  constraint symmetric L6.start L10 L11.end
  constraint symmetric L4.end L10 L12.end
  constraint symmetric L4.start L10 L12.start
  constraint symmetric L7.end L10 L13.start
  constraint symmetric A0 L10 A1
extrude "Extrusion14" cut sketch "Skizze12" against normal blind 3.75 contours A0 | A1 | A2 | A3 | A4 | A5 | A6 | A7 bodies 1
extrude "Extrusion15" cut sketch "Skizze11" against normal blind 3.75 contours A0 | A1 bodies 1
extrude "Extrusion16" cut sketch "Skizze13" against normal blind 2.75 contours L4 L5 L6 L7 L8 L9 L10 L11 L12 L13 L14 L15 | A0 A1 | L21 L22 L23 L24 L25 L26 L27 L28 L29 L30 L31 L32 | A2 A3 | L33 L42 L43 L44 L45 L46 L47 L48 L53 L57 L58 L59 | L36 L37 L38 L40 L41 L49 L52 L55 L56 L61 L62 L64 | A4 A5 | A6 A7 bodies 1
extrude "Extrusion17" cut sketch "Skizze14" against normal blind 2.75 contours L4 L5 L6 L7 L8 L9 | A0 bodies 1
extrude "Extrusion18" cut sketch "Skizze14" against normal blind 11 contours A0 | A1 bodies 1
extrude "Extrusion19" cut sketch "Skizze13" against normal blind 11 contours A0 A1 | A2 A3 | A4 A5 | A6 A7 bodies 1
split "Teilen1" by plane through (0, 0, 0) normal (0, 1, 0) bodies 1 makes body 2 at (14.9879, 54.5943, 0)
split "Teilen2" by plane through (0, 0, 0) normal (1, 0, 0) bodies 1 2 makes body 4 at (32.9453, 53.0912, 0) makes body 3 at (34.2988, -55.9138, 0)
copy_body "Körper->Berechn3" bodies 2 removing the originals makes body 5 in component "BoTech.StarClock.Top.A"
copy_body "Körper->Berechn4" bodies 1 removing the originals makes body 6 in component "BoTech.StarClock.Top.B"
copy_body "Körper->Berechn5" bodies 3 removing the originals makes body 7 in component "BoTech.StarClock.Top.C"
copy_body "Körper->Berechn6" bodies 4 removing the originals makes body 8 in component "BoTech.StarClock.Top.D"
component "BoTech.StarClock.Top.A" placed x (1, 0, 0) y (0, 1, 0) z (0, 0, 1) at (0, 0, 0)
component "BoTech.StarClock.Top.B" placed x (1, 0, 0) y (0, 1, 0) z (0, 0, 1) at (0, 0, 0)
component "BoTech.StarClock.Top.C" placed x (1, 0, 0) y (0, 1, 0) z (0, 0, 1) at (0, 0, 0)
component "BoTech.StarClock.Top.D" placed x (1, 0, 0) y (0, 1, 0) z (0, 0, 1) at (0, 0, 0)
